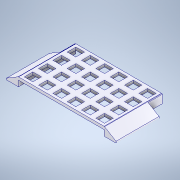
# Autodesk Inventor part: MainPhalange_grip_support
Saved by Autodesk Inventor 2020 (Build 240168000, 168)
## iProperties
Created: 2019-10-16
Part Number: MainPhalange_grip_support
Material: Generic
Document SubType Name: Modeling
Designer: ayad493
Density: 1 g/cm^3
Appearance: Cool White
Author: ayad493
Autodesk Inventor part; units mm, degrees
ref_plane "YZ Plane" through (0, 0, 0) normal (1, 0, 0) x (0, 1, 0)
ref_plane "XZ Plane" through (0, 0, 0) normal (0, 1, 0) x (-1, 0, 0)
ref_plane "XY Plane" through (0, 0, 0) normal (0, 0, 1) x (1, 0, 0)
sketch "Sketch1" plane through (0, 0, 0) normal (0, 0, 1) x (1, 0, 0)
  line L0 (1.0831, 0) -> (38.9169, 0)
  line L1 (40, 0) -> (40, 3)
  line L2 (34.9169, 3) -> (5.0831, 3)
  line L3 (0, 3) -> (0, 0)
  line L4 (0, 0) -> (0, 3)
  line L5 (0, 3) -> (5, 3)
  line L6 (4.9287, 2.9572) -> (0.9287, 0.5572)
  line L7 (40, 3) -> (35, 3)
  line L8 (35.0713, 2.9572) -> (39.0713, 0.5572)
  arc A0 (5.0831, 3) -> (4.9287, 2.9572) centre (5.0831, 2.7) ccw
  arc A1 (0.9287, 0.5572) -> (1.0831, 0) centre (1.0831, 0.3) ccw
  arc A2 (35.0713, 2.9572) -> (34.9169, 3) centre (34.9169, 2.7) ccw
  arc A3 (38.9169, 0) -> (39.0713, 0.5572) centre (38.9169, 0.3) ccw
  dimension "d0" = 40
  dimension "d1" = 3
  dimension "d2" = 5
  dimension "d3" = 5
  dimension "d6" = 0.3
  constraints: 18 end point, 8 point on circle, 8 point on line, 8 tangent, 4 centre point, 3 equal radius, 2 parallel, 2 perpendicular, 1 horizontal
  measures "d0" distance of L3.start L1.end
  measures "d1" distance of L1.end L1.start
  measures "d2" distance of L5.end L3.start
  measures "d3" distance of L7.end L1.end
  measures "d6" radius of A0
extrude "Extrusion1" add sketch "Sketch1" along normal blind 20
sketch "Sketch2" plane through (0, 0, 20) normal (0, 0, 1) x (1, 0, 0)
  line L0 (34.9169, 3) -> (5.0831, 3) projected
  line L1 (5.0831, 3) -> (5.0831, 2)
  line L2 (5.0831, 2) -> (34.9169, 2)
  line L3 (34.9169, 2) -> (34.9169, 3)
  line L4 (5.0831, 2) -> (5.0831, 0)
  line L5 (1.0831, 0) -> (38.9169, 0) projected
  line L6 (34.9169, 2) -> (34.9169, 0)
  line L7 (5.0831, 2) -> (34.9169, 2)
  line L8 (34.9169, 2) -> (34.9169, 0)
  line L9 (34.9169, 0) -> (5.0831, 0)
  line L10 (5.0831, 0) -> (5.0831, 2)
  point P0 (0, 0)
  dimension "d7" = 1
  constraints: 18 end point, 3 perpendicular, 3 vertical, 2 parallel, 1 horizontal, 1 point on line
  measures "d7" distance of L0.end L1.end
extrude "Extrusion2" cut sketch "Sketch2" against normal through all contours L6 L5 L4 L2
sketch "Sketch3" plane through (5.0831, 3, 0) normal (0, 1, 0) x (1, 0, 0)
  line L0 (29.8338, 0) -> (0, 0) projected
  line L1 (0, 0) -> (5, 0)
  line L2 (2.5, 0) -> (2.5, -20)
  line L3 (29.8338, -20) -> (0, -20) projected
  line L4 (2.5, 0) -> (2.5, -5)
  line L5 (1, -4) -> (4, -4)
  line L6 (4, -4) -> (4, -1)
  line L7 (4, -1) -> (1, -1)
  line L8 (1, -1) -> (1, -4)
  line L9 (1, -4) -> (4, -1) construction
  line L10 (4, -4) -> (1, -1) construction
  line L11 (9, -1) -> (6, -1)
  line L12 (9, -4) -> (9, -1)
  line L13 (6, -1) -> (6, -4)
  line L14 (6, -4) -> (9, -4)
  line L15 (14, -1) -> (11, -1)
  line L16 (14, -4) -> (14, -1)
  line L17 (11, -1) -> (11, -4)
  line L18 (11, -4) -> (14, -4)
  line L19 (19, -1) -> (16, -1)
  line L20 (19, -4) -> (19, -1)
  line L21 (16, -1) -> (16, -4)
  line L22 (16, -4) -> (19, -4)
  line L23 (24, -1) -> (21, -1)
  line L24 (24, -4) -> (24, -1)
  line L25 (21, -1) -> (21, -4)
  line L26 (21, -4) -> (24, -4)
  line L27 (29, -1) -> (26, -1)
  line L28 (29, -4) -> (29, -1)
  line L29 (26, -1) -> (26, -4)
  line L30 (26, -4) -> (29, -4)
  line L31 (4, -6) -> (1, -6)
  line L32 (4, -9) -> (4, -6)
  line L33 (1, -6) -> (1, -9)
  line L34 (1, -9) -> (4, -9)
  line L35 (9, -6) -> (6, -6)
  line L36 (9, -9) -> (9, -6)
  line L37 (6, -6) -> (6, -9)
  line L38 (6, -9) -> (9, -9)
  line L39 (14, -6) -> (11, -6)
  line L40 (14, -9) -> (14, -6)
  line L41 (11, -6) -> (11, -9)
  line L42 (11, -9) -> (14, -9)
  line L43 (19, -6) -> (16, -6)
  line L44 (19, -9) -> (19, -6)
  line L45 (16, -6) -> (16, -9)
  line L46 (16, -9) -> (19, -9)
  line L47 (24, -6) -> (21, -6)
  line L48 (24, -9) -> (24, -6)
  line L49 (21, -6) -> (21, -9)
  line L50 (21, -9) -> (24, -9)
  line L51 (29, -6) -> (26, -6)
  line L52 (29, -9) -> (29, -6)
  line L53 (26, -6) -> (26, -9)
  line L54 (26, -9) -> (29, -9)
  line L55 (4, -11) -> (1, -11)
  line L56 (4, -14) -> (4, -11)
  line L57 (1, -11) -> (1, -14)
  line L58 (1, -14) -> (4, -14)
  line L59 (9, -11) -> (6, -11)
  line L60 (9, -14) -> (9, -11)
  line L61 (6, -11) -> (6, -14)
  line L62 (6, -14) -> (9, -14)
  line L63 (14, -11) -> (11, -11)
  line L64 (14, -14) -> (14, -11)
  line L65 (11, -11) -> (11, -14)
  line L66 (11, -14) -> (14, -14)
  line L67 (19, -11) -> (16, -11)
  line L68 (19, -14) -> (19, -11)
  line L69 (16, -11) -> (16, -14)
  line L70 (16, -14) -> (19, -14)
  line L71 (24, -11) -> (21, -11)
  line L72 (24, -14) -> (24, -11)
  line L73 (21, -11) -> (21, -14)
  line L74 (21, -14) -> (24, -14)
  line L75 (29, -11) -> (26, -11)
  line L76 (29, -14) -> (29, -11)
  line L77 (26, -11) -> (26, -14)
  line L78 (26, -14) -> (29, -14)
  line L79 (4, -16) -> (1, -16)
  line L80 (4, -19) -> (4, -16)
  line L81 (1, -16) -> (1, -19)
  line L82 (1, -19) -> (4, -19)
  line L83 (9, -16) -> (6, -16)
  line L84 (9, -19) -> (9, -16)
  line L85 (6, -16) -> (6, -19)
  line L86 (6, -19) -> (9, -19)
  line L87 (14, -16) -> (11, -16)
  line L88 (14, -19) -> (14, -16)
  line L89 (11, -16) -> (11, -19)
  line L90 (11, -19) -> (14, -19)
  line L91 (19, -16) -> (16, -16)
  line L92 (19, -19) -> (19, -16)
  line L93 (16, -16) -> (16, -19)
  line L94 (16, -19) -> (19, -19)
  line L95 (24, -16) -> (21, -16)
  line L96 (24, -19) -> (24, -16)
  line L97 (21, -16) -> (21, -19)
  line L98 (21, -19) -> (24, -19)
  line L99 (29, -16) -> (26, -16)
  line L100 (29, -19) -> (29, -16)
  line L101 (26, -16) -> (26, -19)
  line L102 (26, -19) -> (29, -19)
  point P0 (-5.0831, 0)
  point P1 (2.5, -2.5)
  dimension "d10" = 5
  dimension "d11" = 5
  dimension "d12" = 3
  dimension "d13" = 3
  dimension "d16" = 5
  dimension "d19" = 5
  constraints: 202 end point, 4 midpoint, 3 point on line, 2 horizontal, 2 parallel, 2 vertical, 1 perpendicular, 184 other
  measures "d10" distance of L0.end L1.end
  measures "d11" distance of L2.start L4.end
  measures "d12" distance of L7.end L6.end
  measures "d13" distance of L6.end L5.end
  measures "d16" distance of L6.end L11.start
  measures "d19" distance of L6.end L31.start
extrude "Extrusion3" cut sketch "Sketch3" against normal blind 2
sketch "Sketch4" plane through (38.9169, 0, 0) normal (0, -1, 0) x (1, 0, 0)
  line L0 (-37.8338, 0) -> (-38.1338, 0) projected
  line L1 (-38.1338, 0) -> (-34.1738, 0)
  line L2 (-34.1738, 0) -> (-34.1738, 5)
  line L3 (-34.1738, 5) -> (-38.1338, 5)
  line L4 (-38.1338, 5) -> (-38.1338, 0)
  line L5 (0.3, 0) -> (0.3, 20) projected
  line L6 (0.3, 0) -> (-3.66, 0)
  line L7 (-3.66, 0) -> (-3.66, 5)
  line L8 (-3.66, 5) -> (0.3, 5)
  line L9 (0.3, 5) -> (0.3, 0)
  point P0 (-38.9169, 0)
  point P1 (-37.9882, 0)
  dimension "d24" = 3.96
  dimension "d25" = 5
  dimension "d26" = 3.96
  dimension "d27" = 5
  constraints: 16 end point, 4 parallel, 2 horizontal, 2 perpendicular, 2 point on line
  measures "d24" distance of L3.end L2.end
  measures "d25" distance of L2.end L1.end
  measures "d26" distance of L7.end L8.end
  measures "d27" distance of L6.end L7.end
extrude "Extrusion4" cut sketch "Sketch4" against normal through all
body "Solid1"
